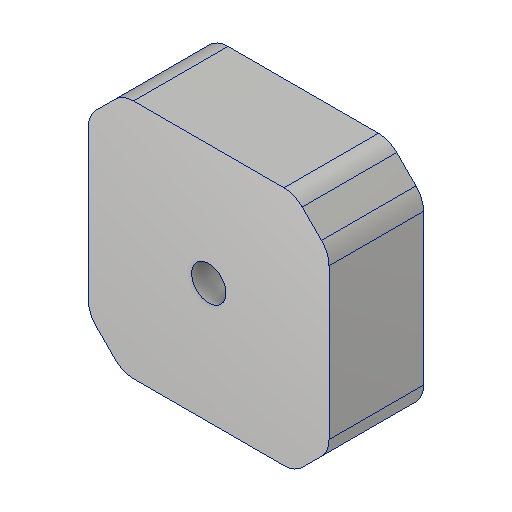
# Autodesk Inventor part: CNCM_ALU_Visual_inspection_tray_leg_holder
Saved by Autodesk Inventor 2025 (Build 290162010, 162A)
## iProperties
Created: 2018-09-18
Part Number: CNCM_ALU_Visual_inspection_tray_leg_holder
Material: Aluminum 6061
Document SubType Name: Modeling
Designer: Andrzej
Density: 2.7 g/cm^3
Appearance: Aluminum - Flat
Mass: 1.82365 g
Surface Area: 7.49266 cm^2
Volume: 0.675425 cm^3
Author: Andrzej
Autodesk Inventor part; units mm, degrees
ref_plane "YZ Plane" through (0, 0, 0) normal (1, 0, 0) x (0, 1, 0)
ref_plane "XZ Plane" through (0, 0, 0) normal (0, 1, 0) x (-1, 0, 0)
ref_plane "XY Plane" through (0, 0, 0) normal (0, 0, 1) x (1, 0, 0)
sketch "Sketch1" plane through (0, 0, 0) normal (0, 0, 1) x (1, 0, 0)
  line L0 (0, 0) -> (8, 0)
  line L1 (8, 0) -> (8, 8)
  line L2 (8, 8) -> (0, 8)
  line L3 (0, 8) -> (0, 0)
  line L4 (-3, 11) -> (11, 11)
  line L5 (11, 11) -> (11, -3)
  line L6 (11, -3) -> (-3, -3)
  line L7 (-3, -3) -> (-3, 11)
  dimension "d0" = 8
  dimension "d1" = 8
  dimension "d2" = 3
  constraints: 16 end point, 4 parallel, 2 perpendicular, 1 horizontal, 3 other
  measures "d0" distance of L2.end L1.end
  measures "d1" distance of L1.end L0.end
  measures "d2" distance between parallel lines of L2 L4
extrude "Extrusion1" add sketch "Sketch1" along normal blind 1.5 contours L3 L2 L1 L0 | L4 L5 L6 L7
extrude "Extrusion2" add sketch "Sketch1" against normal blind 4
chamfer "Chamfer1" distance 2.5 angle 45 4 edges at (8, 4, -4) (4, 0, -4) (4, 8, -4) (0, 4, -4)
sketch "Sketch2" plane through (0, 0, 0) normal (0, 0, -1) x (-1, 0, 0)
  line L0 (-8, 8) -> (-8, 0) projected
  line L1 (-8, 0) -> (0, 0) projected
  line L2 (0, 0) -> (0, 8) projected
  line L3 (0, 8) -> (-8, 8) projected
  point P0 (-4, 4)
hole "Hole1" at (4, 4, 0) direction (0, 0, 1) diameter 2 depth 8 tip angle 118
chamfer "Chamfer2" distance 2 angle 45 8 edges at (9.25, 9.25, -2.75) (-1.25, 9.25, -2.75) (-1.25, -1.25, -2.75) (9.25, -1.25, -2.75) (11, -3, -1.25) (11, 11, -1.25) (-3, -3, -1.25) (-3, 11, -1.25)
fillet "Fillet2" radius 1.5 8 edges at (11, 9, -1.25) (9, 11, -1.25) (11, -1, -1.25) (9, -3, -1.25) (-1, -3, -1.25) (-3, -1, -1.25) (-1, 11, -1.25) (-3, 9, -1.25)
body "Solid1"
